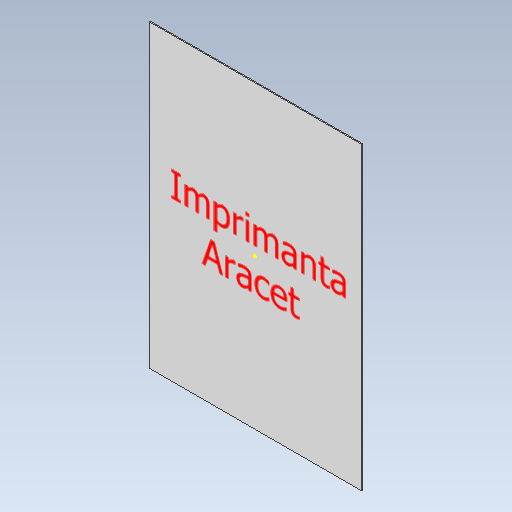
# Autodesk Inventor part: Foaie A4
Saved by Autodesk Inventor 2020 (Build 240168000, 168)
## iProperties
Created: 2020-12-18
Part Number: Foaie A4
Material: Generic
Document SubType Name: Modeling
Designer: Iulian Bors
Density: 1 g/cm^3
Appearance: Default
Author: Iulian Bors
Subject: A4 paper
Autodesk Inventor part; units mm, degrees
ref_plane "YZ Plane" through (0, 0, 0) normal (1, 0, 0) x (0, 1, 0)
ref_plane "XZ Plane" through (0, 0, 0) normal (0, 1, 0) x (-1, 0, 0)
ref_plane "XY Plane" through (0, 0, 0) normal (0, 0, 1) x (1, 0, 0)
sketch "Sketch1" plane through (0, 0, 0) normal (0, 0, 1) x (1, 0, 0)
  line L0 (-105, 148.5) -> (105, 148.5)
  line L1 (105, 148.5) -> (105, -148.5)
  line L2 (105, -148.5) -> (-105, -148.5)
  line L3 (-105, -148.5) -> (-105, 148.5)
  point P0 (0, 0)
  point P1 (0, 148.5)
  point P2 (-105, 0)
  dimension "d0" = 210
  dimension "d1" = 297
  constraints: 8 end point, 2 midpoint, 2 parallel, 1 horizontal, 1 horizontal alignment, 1 perpendicular, 1 vertical alignment
  measures "d0" distance of L1.end L2.end
  measures "d1" distance of L2.end L0.start
extrude "Extrusion1" add sketch "Sketch1" along normal blind 1
sketch "Sketch2" plane through (0, 0, 1) normal (0, 0, 1) x (1, 0, 0)
  line L0 (-85.0261, 33.4604) -> (107.408, 33.4604) construction
  line L1 (107.408, 33.4604) -> (107.408, 25.31) construction
  line L2 (107.408, 25.31) -> (-85.0261, 25.31) construction
  line L3 (-85.0261, 25.31) -> (-85.0261, 33.4604) construction
  point P0 (0, 0)
  dimension "d3" = 0
  constraints: 2 other
body "Solid1"
